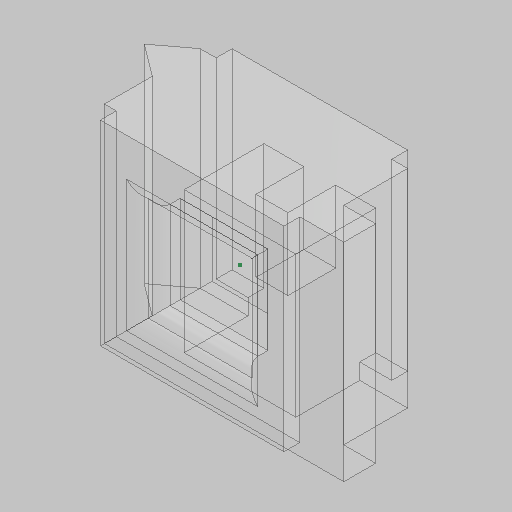
# Autodesk Inventor part: NV_module
Saved by Autodesk Inventor 2026.1 (Build 301233020, 233B)
## iProperties
Created: 2026-01-23
Part Number: NV_module
Material: PET Plastic
Document SubType Name: Modeling
Designer: samuel
Density: 1.541 g/cm^3
Appearance: Polycarbonate - Clear
Author: samuel
Autodesk Inventor part; units mm, degrees
ref_plane "YZ Plane" through (0, 0, 0) normal (1, 0, 0) x (0, 1, 0)
ref_plane "XZ Plane" through (0, 0, 0) normal (0, 1, 0) x (-1, 0, 0)
ref_plane "XY Plane" through (0, 0, 0) normal (0, 0, 1) x (1, 0, 0)
sketch "Sketch1" plane through (0, 0, 0) normal (0, 0, 1) x (1, 0, 0)
  line L0 (-6.5, -6.5) -> (6.5, -6.5)
  line L1 (6.5, -6.5) -> (6.5, 6.5)
  line L2 (6.5, 6.5) -> (-6.5, 6.5)
  line L3 (-6.5, 6.5) -> (-6.5, -6.5)
  line L4 (-6.5, -6.5) -> (6.5, 6.5) construction
  line L5 (6.5, -6.5) -> (-6.5, 6.5) construction
  line L6 (-5.75, -5.75) -> (5.75, -5.75)
  line L7 (5.75, -5.75) -> (5.75, 5.75)
  line L8 (5.75, 5.75) -> (-5.75, 5.75)
  line L9 (-5.75, 5.75) -> (-5.75, -5.75)
  point P0 (0, 0)
  dimension "d0" = 13
  dimension "d1" = 13
  dimension "d2" = 0.75
  constraints: 20 end point, 4 parallel, 2 midpoint, 2 perpendicular, 1 horizontal, 3 other
  measures "d0" distance of L2.end L1.end
  measures "d1" distance of L1.end L0.end
  measures "d2" distance between parallel lines of L3 L9
extrude "Extrusion1" add sketch "Sketch1" along normal blind 7.5 contours L9 L8 L7 L6
extrude "Extrusion2" add sketch "Sketch1" along normal blind 7
sketch "Sketch2" plane through (0, 0, 7.5) normal (0, 0, 1) x (1, 0, 0)
  line L0 (5.75, 5.75) -> (-5.75, 5.75) projected
  line L1 (-5.75, -5.75) -> (5.75, -5.75)
  line L2 (5.75, -5.75) -> (5.75, 5.75)
  line L3 (5.75, 5.75) -> (-5.75, 5.75)
  line L4 (-5.75, 5.75) -> (-5.75, -5.75)
  line L5 (-5.75, -5.75) -> (5.75, 5.75) construction
  line L6 (5.75, -5.75) -> (-5.75, 5.75) construction
  line L7 (-3.75, -3.75) -> (3.75, -3.75)
  line L8 (3.75, -3.75) -> (3.75, 3.75)
  line L9 (3.75, 3.75) -> (-3.75, 3.75)
  line L10 (-3.75, 3.75) -> (-3.75, -3.75)
  line L11 (-4.75, 4.75) -> (4.75, 4.75)
  line L12 (4.75, 4.75) -> (4.75, -4.75)
  line L13 (4.75, -4.75) -> (-4.75, -4.75)
  line L14 (-4.75, -4.75) -> (-4.75, 4.75)
  line L15 (-2.75, 2.75) -> (2.75, 2.75)
  line L16 (2.75, 2.75) -> (2.75, -2.75)
  line L17 (2.75, -2.75) -> (-2.75, -2.75)
  line L18 (-2.75, -2.75) -> (-2.75, 2.75)
  point P0 (0, 0)
  dimension "d7" = 2
  dimension "d10" = 1
  dimension "d14" = 1
  constraints: 36 end point, 8 parallel, 4 perpendicular, 2 midpoint, 1 horizontal, 9 other
  measures "d7" distance between parallel lines of L4 L10
  measures "d10" distance between parallel lines of L9 L11
  measures "d14" distance between parallel lines of L9 L15
extrude "Extrusion3" cut sketch "Sketch2" against normal through all contours L15 L16 L17 L18
sketch "Sketch6" plane through (0, 0, 0) normal (0, 0, -1) x (-1, 0, 0)
  line L0 (2.75, -2.75) -> (2.75, 2.75) projected
  line L1 (-2.75, -2.75) -> (2.75, -2.75)
  line L2 (2.75, -2.75) -> (2.75, 2.75)
  line L3 (2.75, 2.75) -> (-2.75, 2.75)
  line L4 (-2.75, 2.75) -> (-2.75, -2.75)
  line L5 (-2.75, -2.75) -> (2.75, 2.75) construction
  line L6 (2.75, -2.75) -> (-2.75, 2.75) construction
  line L7 (-3.75, 3.75) -> (3.75, 3.75)
  line L8 (3.75, 3.75) -> (3.75, -3.75)
  line L9 (3.75, -3.75) -> (-3.75, -3.75)
  line L10 (-3.75, -3.75) -> (-3.75, 3.75)
  line L11 (6.5, -6.5) -> (-6.5, -6.5) projected
  line L12 (-3.75, -3.75) -> (3.75, -3.75)
  line L13 (3.75, -3.75) -> (3.75, -6.5)
  line L14 (3.75, -6.5) -> (-3.75, -6.5)
  line L15 (-3.75, -6.5) -> (-3.75, -3.75)
  line L16 (-1.75, 1.75) -> (1.75, 1.75)
  line L17 (1.75, 1.75) -> (1.75, -1.75)
  line L18 (1.75, -1.75) -> (-1.75, -1.75)
  line L19 (-1.75, -1.75) -> (-1.75, 1.75)
  point P0 (0, 0)
  dimension "d25" = 1
  dimension "d36" = 1
  constraints: 36 end point, 8 parallel, 4 perpendicular, 2 horizontal, 2 midpoint, 1 point on line, 6 other
  measures "d25" distance between parallel lines of L3 L7
  measures "d36" distance between parallel lines of L3 L16
extrude "Extrusion9" add sketch "Sketch6" against normal blind 6 contours L1 L4 L3 L0
sketch "Sketch7" plane through (0, 0, 0) normal (0, 0, -1) x (-1, 0, 0)
  line L0 (6.5, -6.5) -> (-6.5, -6.5) projected
  line L1 (-3.5, -6.5) -> (3.5, -6.5)
  line L2 (3.5, -6.5) -> (3.5, 2.35)
  line L3 (3.5, 2.35) -> (-3.5, 2.35)
  line L4 (-3.5, 2.35) -> (-3.5, -6.5)
  line L5 (-6.5, -6.5) -> (-6.5, 6.5) projected
  line L6 (6.5, 6.5) -> (6.5, -6.5) projected
  line L7 (-1.75, 1.75) -> (1.75, 1.75) projected
  point P0 (0, 0)
  dimension "d47" = 3
  dimension "d48" = 3
  dimension "d49" = 0.6
  constraints: 8 end point, 2 parallel, 1 horizontal, 1 perpendicular, 1 point on line
  measures "d47" distance between parallel lines of L5 L4
  measures "d48" distance between parallel lines of L6 L2
  measures "d49" distance between parallel lines of L3 L7
extrude "Extrusion10" cut sketch "Sketch7" against normal blind 5
chamfer "Chamfer5" distance 1 angle 45 4 edges at (-1.75, 0, 6) (0, -1.75, 6) (1.75, 0, 6) (0, 1.75, 6)
sketch "Sketch8" plane through (0, 0, 5) normal (0, 0, -1) x (-1, 0, 0)
  point P0 (0, 0)
sketch "Sketch9" plane through (0, 0, 0) normal (0, 0, -1) x (-1, 0, 0)
  line L0 (-6.5, 6.5) -> (6.5, 6.5) projected
  line L1 (6.5, 6.5) -> (6.5, -6.5) projected
  line L2 (-6.5, 6.5) -> (6.5, 6.5)
  line L3 (6.5, 6.5) -> (6.5, -6.5)
  line L4 (6.5, -6.5) -> (-6.5, -6.5)
  line L5 (-6.5, -6.5) -> (-6.5, 6.5)
  line L6 (-5.5, 5.5) -> (5.5, 5.5)
  line L7 (5.5, 5.5) -> (5.5, -5.5)
  line L8 (5.5, -5.5) -> (-5.5, -5.5)
  line L9 (-5.5, -5.5) -> (-5.5, 5.5)
  point P0 (0, 0)
  dimension "d50" = 1
  constraints: 16 end point, 4 parallel, 2 perpendicular, 1 horizontal, 3 other
  measures "d50" distance between parallel lines of L5 L9
extrude "Extrusion11" cut sketch "Sketch9" against normal blind 1
sketch "Sketch10" plane through (-3.5, 2.35, 0) normal (0, -1, 0) x (1, 0, 0)
  line L0 (-2, 0) -> (9, 0) projected
  line L1 (4.5, 3) -> (2.5, 3)
  line L2 (2.5, 3) -> (2.5, 0)
  line L3 (2.5, 0) -> (4.5, 0)
  line L4 (4.5, 0) -> (4.5, 3)
  point P0 (3.5, 0)
  point P1 (3.5, 0)
  point P2 (4.5, 0)
  dimension "d53" = 3
  dimension "d54" = 2
  dimension "d55" = 1
  constraints: 8 end point, 2 parallel, 1 horizontal, 1 midpoint, 1 perpendicular, 1 point on line
  measures "d53" distance of L3.end L1.start
  measures "d54" distance of L1.start L1.end
  measures "d55" distance from line of point (3.5, 0) L4
extrude "Extrusion12" add sketch "Sketch10" along normal blind 4.5
sketch "Sketch11" plane through (-6.5, 6.5, 7) normal (0, 1, 0) x (1, 0, 0)
  line L0 (13, 6) -> (13, 0) projected
  line L1 (13, 0) -> (15, 0)
  line L2 (15, 0) -> (15, 2)
  line L3 (15, 2) -> (13, 2)
  line L4 (13, 2) -> (13, 0)
  line L5 (0, 6) -> (0, 0) projected
  line L6 (0, 6) -> (0, 3)
  line L7 (0, 4.5) -> (-2, 4.5)
  line L8 (-2, 4.5) -> (0, 3)
  line L9 (-2, 4.5) -> (0, 6)
  point P0 (6.5, 7)
  point P1 (13, 2)
  dimension "d58" = 2
  dimension "d59" = 2
  dimension "d60" = 2
  constraints: 16 end point, 2 horizontal, 2 midpoint, 2 parallel, 1 perpendicular
  measures "d58" distance of L3.end L2.end
  measures "d59" distance of L2.end L1.end
  measures "d60" distance of L7.start L7.end
extrude "Extrusion13" add sketch "Sketch11" against normal blind 13
sketch "Sketch12" plane through (-5.5, 5.5, 0) normal (0, 1, 0) x (1, 0, 0)
  line L0 (0, 0) -> (11, 0)
  line L1 (11, 0) -> (11, -7.4478)
  line L2 (11, -7.4478) -> (0, -7.4478)
  line L3 (0, -7.4478) -> (0, 0)
  line L4 (-0.25, -7.5) -> (11.25, -7.5) projected
  line L5 (0, 0) -> (11, 0)
  line L6 (11, 0) -> (11, -7.5)
  line L7 (11, -7.5) -> (0, -7.5)
  line L8 (0, -7.5) -> (0, 0)
  point P0 (5.5, 0)
  constraints: 16 end point, 4 parallel, 2 horizontal, 2 perpendicular, 1 point on line
extrude "Extrusion14" add sketch "Sketch12" along normal blind 1
sketch "Sketch13" plane through (0, 0, 7.5) normal (0, 0, 1) x (1, 0, 0)
  line L0 (5.75, 5.75) -> (5.5, 5.75) projected
  line L1 (-5.5, 6.5) -> (-5.5, -5.5) projected
  line L2 (5.5, 5.75) -> (-5.5, 5.75)
  line L3 (-5.5, 5.75) -> (-5.5, -5.5)
  line L4 (-5.5, -5.5) -> (5.5, -5.5)
  line L5 (5.5, -5.5) -> (5.5, 5.75)
  line L6 (5.75, -5.75) -> (-5.75, -5.75)
  line L7 (-5.75, -5.75) -> (-5.75, 6)
  line L8 (-5.75, 6) -> (5.75, 6)
  line L9 (5.75, 6) -> (5.75, -5.75)
  point P0 (0, 0)
  point P1 (-5.5, 6)
  constraints: 16 end point, 4 parallel, 2 perpendicular, 1 horizontal, 3 other
extrude "Extrusion15" cut sketch "Sketch13" against normal blind 0.5 contours L9 L6 L7 L8 L1 L4 L5 L0
sketch "Sketch14" plane through (0, 0, 7.5) normal (0, 0, 1) x (1, 0, 0)
  line L0 (5.5, 6.5) -> (-5.5, 6.5) projected
  line L1 (-5.5, 6.5) -> (5.5, 6.5)
  line L2 (5.5, 6.5) -> (5.5, -5.5)
  line L3 (5.5, -5.5) -> (-5.5, -5.5)
  line L4 (-5.5, -5.5) -> (-5.5, 6.5)
  line L5 (-3.25, 3.25) -> (-3.25, -3.25) projected
  line L6 (-3.25, -3.25) -> (3.25, -3.25) projected
  line L7 (-3.25, 3.25) -> (3.25, 3.25)
  line L8 (3.25, 3.25) -> (3.25, -3.25)
  line L9 (3.25, -3.25) -> (-3.25, -3.25)
  line L10 (-3.25, -3.25) -> (-3.25, 3.25)
  point P0 (0, 0)
  constraints: 16 end point, 4 parallel, 2 horizontal, 2 perpendicular
extrude "Extrusion16" add sketch "Sketch14" along normal blind 0.5
sketch "Sketch15" plane through (0, 0, 7) normal (0, 0, 1) x (1, 0, 0)
  line L0 (5.5, 6.5) -> (5.5, -5.5) projected
  line L1 (5.5, 6.5) -> (-5.5, 6.5)
  line L2 (-5.5, 6.5) -> (-5.5, -5.5)
  line L3 (-5.5, -5.5) -> (5.5, -5.5)
  line L4 (5.5, -5.5) -> (5.5, 6.5)
  line L5 (5.75, -5.75) -> (-5.75, -5.75)
  line L6 (-5.75, -5.75) -> (-5.75, 6.75)
  line L7 (-5.75, 6.75) -> (5.75, 6.75)
  line L8 (5.75, 6.75) -> (5.75, -5.75)
  line L9 (5.75, 6.5) -> (-5.75, 6.5)
  point P0 (0, 0)
  dimension "d69" = 0.25
  constraints: 18 end point, 4 parallel, 3 perpendicular, 2 point on line, 1 horizontal, 3 other
  measures "d69" distance between parallel lines of L3 L5
extrude "Extrusion17" add sketch "Sketch15" along normal blind 1 contours L9 L8 L5 L6 L2 L3 L0
fillet "Fillet1" radius 1 8 edges at (0, 2.75, 7.5) (2.75, 0, 7.5) (-2.75, 0, 7.5) (0, -2.75, 7.5) (0, 3.25, 8) (-3.25, 0, 8) (0, -3.25, 8) (3.25, 0, 8)
body "Solid1"
